Autodesk Inventor part; units mm, degrees
(part 2 of 2)
  line L320 (-21.6501, 50.3257) -> (-21.6501, 48.006)
  line L321 (-22.7741, 46.882) -> (-22.7741, 51.4497)
  line L322 (-19.4696, 52.5096) -> (-19.4696, 51.4497)
  line L323 (-13.5344, 50.3565) -> (-13.5344, 48.0368)
  line L324 (-15.3794, 53.4802) -> (-9.591, 53.4802)
  line L325 (-11.2436, 52.5096) -> (-11.2436, 51.4805)
  line L326 (-17.5447, 51.4497) -> (-17.5447, 46.882)
  line L327 (-14.6585, 46.9128) -> (-14.6585, 51.4805)
  line L328 (-14.6585, 51.4805) -> (-12.4852, 51.4805)
  line L329 (-12.4852, 51.4805) -> (-12.4852, 52.5096)
  line L330 (-9.591, 53.4802) -> (-9.591, 52.5096)
  line L331 (-9.591, 52.5096) -> (-11.2436, 52.5096)
  line L332 (-10.5531, 50.3565) -> (-13.5344, 50.3565)
  line L333 (-11.2436, 51.4805) -> (-9.429, 51.4805)
  line L334 (-13.5344, 48.0368) -> (-10.5531, 48.0368)
  line L335 (-9.429, 46.9128) -> (-14.6585, 46.9128)
  line L336 (-9.429, 51.4805) -> (-9.429, 46.9128)
  line L337 (-10.5531, 48.0368) -> (-10.5531, 50.3565)
  line L338 (-88.5687, 43.9647) -> (-88.5687, 42.994)
  line L339 (-88.5687, 42.994) -> (-86.5536, 42.994)
  line L340 (-92.6408, 44.9353) -> (-85.6563, 44.9353)
  line L341 (-87.6776, 41.87) -> (-90.659, 41.87)
  line L342 (-91.783, 42.994) -> (-89.7466, 42.994)
  line L343 (-87.6776, 39.5503) -> (-87.6776, 41.87)
  line L344 (-86.5536, 42.994) -> (-86.5536, 38.4263)
  line L345 (-90.659, 41.87) -> (-90.659, 39.5503)
  line L346 (-90.659, 39.5503) -> (-87.6776, 39.5503)
  line L347 (-86.5536, 38.4263) -> (-91.783, 38.4263)
  line L348 (-91.783, 38.4263) -> (-91.783, 42.994)
  line L349 (-89.7466, 42.994) -> (-89.7466, 43.9647)
  line L350 (-87.5813, 50.5629) -> (-82.3518, 50.5629)
  line L351 (-83.4759, 49.4389) -> (-86.4572, 49.4389)
  line L352 (-86.4572, 49.4389) -> (-86.4572, 47.1192)
  line L353 (-85.6563, 45.9951) -> (-87.5813, 45.9951)
  line L354 (-86.4572, 47.1192) -> (-83.4759, 47.1192)
  line L355 (-81.6326, 43.9647) -> (-88.5687, 43.9647)
  line L356 (-84.5732, 45.9951) -> (-84.5732, 44.9353)
  line L357 (-81.6326, 44.9353) -> (-81.6326, 43.9647)
  line L358 (-84.5732, 44.9353) -> (-81.6326, 44.9353)
  line L359 (-82.3518, 45.9951) -> (-84.5732, 45.9951)
  line L360 (-83.4759, 47.1192) -> (-83.4759, 49.4389)
  line L361 (-82.3518, 50.5629) -> (-82.3518, 45.9951)
  line L362 (-85.6563, 44.9353) -> (-85.6563, 45.9951)
  line L363 (-91.5915, 47.0884) -> (-91.5915, 49.4081)
  line L364 (-89.7466, 43.9647) -> (-95.535, 43.9647)
  line L365 (-93.8823, 44.9353) -> (-93.8823, 45.9644)
  line L366 (-87.5813, 45.9951) -> (-87.5813, 50.5629)
  line L367 (-90.4675, 50.5321) -> (-90.4675, 45.9644)
  line L368 (-90.4675, 45.9644) -> (-92.6408, 45.9644)
  line L369 (-92.6408, 45.9644) -> (-92.6408, 44.9353)
  line L370 (-95.535, 43.9647) -> (-95.535, 44.9353)
  line L371 (-95.535, 44.9353) -> (-93.8823, 44.9353)
  line L372 (-94.5729, 47.0884) -> (-91.5915, 47.0884)
  line L373 (-93.8823, 45.9644) -> (-95.6969, 45.9644)
  line L374 (-91.5915, 49.4081) -> (-94.5729, 49.4081)
  line L375 (-95.6969, 50.5321) -> (-90.4675, 50.5321)
  line L376 (-95.6969, 45.9644) -> (-95.6969, 50.5321)
  line L377 (-94.5729, 49.4081) -> (-94.5729, 47.0884)
  line L378 (-45.9553, 42.018) -> (-40.7259, 42.018)
  line L379 (-41.8499, 40.894) -> (-44.8313, 40.894)
  line L380 (-44.8313, 40.894) -> (-44.8313, 38.5743)
  line L381 (-44.8313, 38.5743) -> (-41.8499, 38.5743)
  line L382 (-40.7259, 42.018) -> (-40.7259, 37.4503)
  line L383 (-45.9553, 37.4503) -> (-45.9553, 42.018)
  line L384 (-44.0304, 37.4503) -> (-45.9553, 37.4503)
  line L385 (-40.7259, 37.4503) -> (-42.9473, 37.4503)
  line L386 (-51.0148, 36.3904) -> (-44.0304, 36.3904)
  line L387 (-42.9473, 37.4503) -> (-42.9473, 36.3904)
  line L388 (-42.9473, 36.3904) -> (-40.0067, 36.3904)
  line L389 (-44.0304, 36.3904) -> (-44.0304, 37.4503)
  line L390 (-40.0067, 35.4198) -> (-46.9428, 35.4198)
  line L391 (-40.0067, 36.3904) -> (-40.0067, 35.4198)
  line L392 (-41.8499, 38.5743) -> (-41.8499, 40.894)
  line L393 (-48.8415, 37.4195) -> (-51.0148, 37.4195)
  line L394 (-51.0148, 37.4195) -> (-51.0148, 36.3904)
  line L395 (-48.1206, 35.4198) -> (-53.909, 35.4198)
  line L396 (-52.2564, 36.3904) -> (-52.2564, 37.4195)
  line L397 (-53.909, 35.4198) -> (-53.909, 36.3904)
  line L398 (-53.909, 36.3904) -> (-52.2564, 36.3904)
  line L399 (-52.9469, 38.5435) -> (-49.9656, 38.5435)
  line L400 (-52.2564, 37.4195) -> (-54.071, 37.4195)
  line L401 (-49.9656, 38.5435) -> (-49.9656, 40.8632)
  line L402 (-48.8415, 41.9872) -> (-48.8415, 37.4195)
  line L403 (-49.9656, 40.8632) -> (-52.9469, 40.8632)
  line L404 (-52.9469, 40.8632) -> (-52.9469, 38.5435)
  line L405 (-54.071, 41.9872) -> (-48.8415, 41.9872)
  line L406 (-54.071, 37.4195) -> (-54.071, 41.9872)
  line L407 (-44.9276, 29.8814) -> (-50.157, 29.8814)
  line L408 (-49.033, 31.0054) -> (-46.0516, 31.0054)
  line L409 (-46.0516, 31.0054) -> (-46.0516, 33.3251)
  line L410 (-44.9276, 34.4492) -> (-44.9276, 29.8814)
  line L411 (-46.9428, 34.4492) -> (-44.9276, 34.4492)
  line L412 (-46.0516, 33.3251) -> (-49.033, 33.3251)
  line L413 (-49.033, 33.3251) -> (-49.033, 31.0054)
  line L414 (-46.9428, 35.4198) -> (-46.9428, 34.4492)
  line L415 (-50.157, 29.8814) -> (-50.157, 34.4492)
  line L416 (-48.1206, 34.4492) -> (-48.1206, 35.4198)
  line L417 (-50.157, 34.4492) -> (-48.1206, 34.4492)
  line L418 (-14.9833, 42.018) -> (-9.7539, 42.018)
  line L419 (-10.8779, 40.894) -> (-13.8593, 40.894)
  line L420 (-13.8593, 40.894) -> (-13.8593, 38.5743)
  line L421 (-13.8593, 38.5743) -> (-10.8779, 38.5743)
  line L422 (-9.7539, 42.018) -> (-9.7539, 37.4503)
  line L423 (-14.9833, 37.4503) -> (-14.9833, 42.018)
  line L424 (-13.0584, 37.4503) -> (-14.9833, 37.4503)
  line L425 (-9.7539, 37.4503) -> (-11.9752, 37.4503)
  line L426 (-20.0428, 36.3904) -> (-13.0584, 36.3904)
  line L427 (-11.9752, 37.4503) -> (-11.9752, 36.3904)
  line L428 (-11.9752, 36.3904) -> (-9.0346, 36.3904)
  line L429 (-13.0584, 36.3904) -> (-13.0584, 37.4503)
  line L430 (-9.0346, 35.4198) -> (-15.9708, 35.4198)
  line L431 (-9.0346, 36.3904) -> (-9.0346, 35.4198)
  line L432 (-10.8779, 38.5743) -> (-10.8779, 40.894)
  line L433 (-17.8695, 37.4195) -> (-20.0428, 37.4195)
  line L434 (-20.0428, 37.4195) -> (-20.0428, 36.3904)
  line L435 (-17.1486, 35.4198) -> (-22.937, 35.4198)
  line L436 (-21.2844, 36.3904) -> (-21.2844, 37.4195)
  line L437 (-22.937, 35.4198) -> (-22.937, 36.3904)
  line L438 (-22.937, 36.3904) -> (-21.2844, 36.3904)
  line L439 (-21.9749, 38.5435) -> (-18.9936, 38.5435)
  line L440 (-21.2844, 37.4195) -> (-23.099, 37.4195)
  line L441 (-18.9936, 38.5435) -> (-18.9936, 40.8632)
  line L442 (-17.8695, 41.9872) -> (-17.8695, 37.4195)
  line L443 (-18.9936, 40.8632) -> (-21.9749, 40.8632)
  line L444 (-21.9749, 40.8632) -> (-21.9749, 38.5435)
  line L445 (-23.099, 41.9872) -> (-17.8695, 41.9872)
  line L446 (-23.099, 37.4195) -> (-23.099, 41.9872)
  line L447 (-13.9556, 29.8814) -> (-19.185, 29.8814)
  line L448 (-18.061, 31.0054) -> (-15.0796, 31.0054)
  line L449 (-15.0796, 31.0054) -> (-15.0796, 33.3251)
  line L450 (-13.9556, 34.4492) -> (-13.9556, 29.8814)
  line L451 (-15.9708, 34.4492) -> (-13.9556, 34.4492)
  line L452 (-15.0796, 33.3251) -> (-18.061, 33.3251)
  line L453 (-18.061, 33.3251) -> (-18.061, 31.0054)
  line L454 (-15.9708, 35.4198) -> (-15.9708, 34.4492)
  line L455 (-19.185, 29.8814) -> (-19.185, 34.4492)
  line L456 (-17.1486, 34.4492) -> (-17.1486, 35.4198)
  line L457 (-19.185, 34.4492) -> (-17.1486, 34.4492)
  line L458 (-31.75, 0) -> (-63.5, 0) construction
  line L459 (-31.75, 88.9) -> (0, 88.9) construction
  line L460 (-31.75, 0) -> (-31.75, 88.9) construction
  line L461 (-24.2924, 69.3883) -> (-29.5218, 69.3883)
  line L462 (-28.3978, 70.5123) -> (-25.4164, 70.5123)
  line L463 (-25.4164, 72.832) -> (-28.3978, 72.832)
  line L464 (-25.4164, 70.5123) -> (-25.4164, 72.832)
  line L465 (-26.2173, 73.956) -> (-24.2924, 73.956)
  line L466 (-24.2924, 73.956) -> (-24.2924, 69.3883)
  line L467 (-29.5218, 69.3883) -> (-29.5218, 73.956)
  line L468 (-29.5218, 73.956) -> (-27.3004, 73.956)
  line L469 (-28.3978, 72.832) -> (-28.3978, 70.5123)
  line L470 (-26.2173, 75.0159) -> (-26.2173, 73.956)
  line L471 (-27.3004, 73.956) -> (-27.3004, 75.0159)
  line L472 (-27.3004, 75.0159) -> (-30.241, 75.0159)
  line L473 (-30.241, 75.0159) -> (-30.241, 75.9864)
  line L474 (-23.3049, 75.9864) -> (-23.3049, 76.9571)
  line L475 (-23.3049, 76.9571) -> (-25.3201, 76.9571)
  line L476 (-30.241, 75.9864) -> (-23.3049, 75.9864)
  line L477 (-17.9913, 75.0159) -> (-17.9913, 73.9868)
  line L478 (-20.2821, 72.8628) -> (-20.2821, 70.5431)
  line L479 (-22.127, 75.9864) -> (-16.3387, 75.9864)
  line L480 (-16.3387, 75.9864) -> (-16.3387, 75.0159)
  line L481 (-16.3387, 75.0159) -> (-17.9913, 75.0159)
  line L482 (-17.3007, 72.8628) -> (-20.2821, 72.8628)
  line L483 (-21.4061, 69.4191) -> (-21.4061, 73.9868)
  line L484 (-17.3007, 70.5431) -> (-17.3007, 72.8628)
  line L485 (-20.2821, 70.5431) -> (-17.3007, 70.5431)
  line L486 (-16.1767, 69.4191) -> (-21.4061, 69.4191)
  line L487 (-16.1767, 73.9868) -> (-16.1767, 69.4191)
  line L488 (-17.9913, 73.9868) -> (-16.1767, 73.9868)
  line L489 (-25.3201, 81.5249) -> (-20.0906, 81.5249)
  line L490 (-20.0906, 81.5249) -> (-20.0906, 76.9571)
  line L491 (-25.3201, 76.9571) -> (-25.3201, 81.5249)
  line L492 (-21.2147, 80.4009) -> (-24.196, 80.4009)
  line L493 (-24.196, 80.4009) -> (-24.196, 78.0812)
  line L494 (-24.196, 78.0812) -> (-21.2147, 78.0812)
  line L495 (-21.2147, 78.0812) -> (-21.2147, 80.4009)
  line L496 (-19.2329, 73.9868) -> (-19.2329, 75.0159)
  line L497 (-21.4061, 73.9868) -> (-19.2329, 73.9868)
  line L498 (-22.127, 76.9571) -> (-22.127, 75.9864)
  line L499 (-20.0906, 76.9571) -> (-22.127, 76.9571)
  line L500 (-19.2329, 75.0159) -> (-26.2173, 75.0159)
  line L501 (-38.0615, 19.4598) -> (-32.8321, 19.4598)
  line L502 (-33.9561, 18.3357) -> (-36.9375, 18.3357)
  line L503 (-36.9375, 18.3357) -> (-36.9375, 16.0161)
  line L504 (-36.9375, 16.0161) -> (-33.9561, 16.0161)
  line L505 (-32.8321, 19.4598) -> (-32.8321, 14.892)
  line L506 (-38.0615, 14.892) -> (-38.0615, 19.4598)
  line L507 (-36.1366, 14.892) -> (-38.0615, 14.892)
  line L508 (-32.8321, 14.892) -> (-35.0534, 14.892)
  line L509 (-43.121, 13.8322) -> (-36.1366, 13.8322)
  line L510 (-35.0534, 14.892) -> (-35.0534, 13.8322)
  line L511 (-35.0534, 13.8322) -> (-32.1128, 13.8322)
  line L512 (-36.1366, 13.8322) -> (-36.1366, 14.892)
  line L513 (-32.1128, 12.8616) -> (-39.0489, 12.8616)
  line L514 (-32.1128, 13.8322) -> (-32.1128, 12.8616)
  line L515 (-33.9561, 16.0161) -> (-33.9561, 18.3357)
  line L516 (-40.9477, 14.8613) -> (-43.121, 14.8613)
  line L517 (-43.121, 14.8613) -> (-43.121, 13.8322)
  line L518 (-40.2268, 12.8616) -> (-46.0152, 12.8616)
  line L519 (-44.3625, 13.8322) -> (-44.3625, 14.8613)
  line L520 (-46.0152, 12.8616) -> (-46.0152, 13.8322)
  line L521 (-46.0152, 13.8322) -> (-44.3625, 13.8322)
  line L522 (-45.0531, 15.9853) -> (-42.0717, 15.9853)
  line L523 (-44.3625, 14.8613) -> (-46.1771, 14.8613)
  line L524 (-42.0717, 15.9853) -> (-42.0717, 18.305)
  line L525 (-40.9477, 19.429) -> (-40.9477, 14.8613)
  line L526 (-42.0717, 18.305) -> (-45.0531, 18.305)
  line L527 (-45.0531, 18.305) -> (-45.0531, 15.9853)
  line L528 (-46.1771, 19.429) -> (-40.9477, 19.429)
  line L529 (-46.1771, 14.8613) -> (-46.1771, 19.429)
  line L530 (-37.0338, 7.3232) -> (-42.2632, 7.3232)
  line L531 (-41.1392, 8.4472) -> (-38.1578, 8.4472)
  line L532 (-38.1578, 8.4472) -> (-38.1578, 10.7669)
  line L533 (-37.0338, 11.8909) -> (-37.0338, 7.3232)
  line L534 (-39.0489, 11.8909) -> (-37.0338, 11.8909)
  line L535 (-38.1578, 10.7669) -> (-41.1392, 10.7669)
  line L536 (-41.1392, 10.7669) -> (-41.1392, 8.4472)
  line L537 (-39.0489, 12.8616) -> (-39.0489, 11.8909)
  line L538 (-42.2632, 7.3232) -> (-42.2632, 11.8909)
  line L539 (-40.2268, 11.8909) -> (-40.2268, 12.8616)
  line L540 (-42.2632, 11.8909) -> (-40.2268, 11.8909)
  line L541 (-22.4246, 19.4981) -> (-17.1952, 19.4981)
  line L542 (-18.3192, 18.3741) -> (-21.3006, 18.3741)
  line L543 (-21.3006, 18.3741) -> (-21.3006, 16.0544)
  line L544 (-21.3006, 16.0544) -> (-18.3192, 16.0544)
  line L545 (-17.1952, 19.4981) -> (-17.1952, 14.9304)
  line L546 (-22.4246, 14.9304) -> (-22.4246, 19.4981)
  line L547 (-20.4997, 14.9304) -> (-22.4246, 14.9304)
  line L548 (-17.1952, 14.9304) -> (-19.4165, 14.9304)
  line L549 (-27.4841, 13.8705) -> (-20.4997, 13.8705)
  line L550 (-19.4165, 14.9304) -> (-19.4165, 13.8705)
  line L551 (-19.4165, 13.8705) -> (-16.4759, 13.8705)
  line L552 (-20.4997, 13.8705) -> (-20.4997, 14.9304)
  line L553 (-16.4759, 12.9) -> (-23.412, 12.9)
  line L554 (-16.4759, 13.8705) -> (-16.4759, 12.9)
  line L555 (-18.3192, 16.0544) -> (-18.3192, 18.3741)
  line L556 (-25.3108, 14.8996) -> (-27.4841, 14.8996)
  line L557 (-27.4841, 14.8996) -> (-27.4841, 13.8705)
  line L558 (-24.5899, 12.9) -> (-30.3783, 12.9)
  line L559 (-28.7257, 13.8705) -> (-28.7257, 14.8996)
  line L560 (-30.3783, 12.9) -> (-30.3783, 13.8705)
  line L561 (-30.3783, 13.8705) -> (-28.7257, 13.8705)
  line L562 (-29.4162, 16.0236) -> (-26.4349, 16.0236)
  line L563 (-28.7257, 14.8996) -> (-30.5403, 14.8996)
  line L564 (-26.4349, 16.0236) -> (-26.4349, 18.3433)
  line L565 (-25.3108, 19.4673) -> (-25.3108, 14.8996)
  line L566 (-26.4349, 18.3433) -> (-29.4162, 18.3433)
  line L567 (-29.4162, 18.3433) -> (-29.4162, 16.0236)
  line L568 (-30.5403, 19.4673) -> (-25.3108, 19.4673)
  line L569 (-30.5403, 14.8996) -> (-30.5403, 19.4673)
  line L570 (-21.3969, 7.3615) -> (-26.6263, 7.3615)
  line L571 (-25.5023, 8.4855) -> (-22.5209, 8.4855)
  line L572 (-22.5209, 8.4855) -> (-22.5209, 10.8052)
  line L573 (-21.3969, 11.9293) -> (-21.3969, 7.3615)
  line L574 (-23.412, 11.9293) -> (-21.3969, 11.9293)
  line L575 (-22.5209, 10.8052) -> (-25.5023, 10.8052)
  line L576 (-25.5023, 10.8052) -> (-25.5023, 8.4855)
  line L577 (-23.412, 12.9) -> (-23.412, 11.9293)
  line L578 (-26.6263, 7.3615) -> (-26.6263, 11.9293)
  line L579 (-24.5899, 11.9293) -> (-24.5899, 12.9)
  line L580 (-26.6263, 11.9293) -> (-24.5899, 11.9293)
  line L581 (-54.8737, 75.3003) -> (-59.8302, 75.3003)
  line L582 (-59.8302, 75.3003) -> (-59.8302, 76.3377)
  line L583 (-59.8302, 76.3377) -> (-57.9859, 76.3377)
  line L584 (-57.9859, 76.3377) -> (-57.9859, 83.1467)
  line L585 (-57.9859, 83.1467) -> (-59.8302, 83.1467)
  line L586 (-59.8302, 83.1467) -> (-59.8302, 84.0771)
  spline S0 degree 2 poles (-59.8302, 84.0771) (-58.7846, 84.0771) (-57.7966, 84.6699) (-57.7307, 85.4932) knots 0 0 0 1 2 2 2
  line L587 (-57.7307, 85.4932) -> (-56.6768, 85.4932)
  line L588 (-56.6768, 85.4932) -> (-56.6768, 76.3377)
  line L589 (-56.6768, 76.3377) -> (-54.8737, 76.3377)
  line L590 (-54.8737, 76.3377) -> (-54.8737, 75.3003)
  spline S1 degree 2 poles (-46.6815, 80.3803) (-46.6815, 77.6468) (-48.2705, 75.0862) (-49.9255, 75.0862) knots 0 0 0 1 2 2 2
  spline S2 degree 2 poles (-49.9255, 75.0862) (-51.6051, 75.0862) (-53.1776, 77.6962) (-53.1776, 80.3721) knots 0 0 0 1 2 2 2
  spline S3 degree 2 poles (-53.1776, 80.3721) (-53.1776, 83.122) (-51.5886, 85.6661) (-49.9255, 85.6661) knots 0 0 0 1 2 2 2
  spline S4 degree 2 poles (-49.9255, 85.6661) (-48.2541, 85.6661) (-46.6815, 83.0314) (-46.6815, 80.3803) knots 0 0 0 1 2 2 2
  spline S5 degree 2 poles (-48.427, 77.2845) (-48.2294, 77.7868) (-48.0647, 79.3347) (-48.0647, 80.3803) knots 0 0 0 1 2 2 2
  spline S6 degree 2 poles (-48.0647, 80.3803) (-48.0647, 81.4259) (-48.2294, 82.9656) (-48.4352, 83.4843) knots 0 0 0 1 2 2 2
  spline S7 degree 2 poles (-48.4352, 83.4843) (-48.641, 84.003) (-49.3573, 84.5382) (-49.9255, 84.5382) knots 0 0 0 1 2 2 2
  spline S8 degree 2 poles (-49.9255, 84.5382) (-50.4936, 84.5382) (-51.2263, 84.003) (-51.4404, 83.4678) knots 0 0 0 1 2 2 2
  spline S9 degree 2 poles (-51.4404, 83.4678) (-51.6462, 82.9491) (-51.7944, 81.3683) (-51.7944, 80.3721) knots 0 0 0 1 2 2 2
  spline S10 degree 2 poles (-51.7944, 80.3721) (-51.7944, 79.3017) (-51.6627, 77.8691) (-51.4486, 77.3092) knots 0 0 0 1 2 2 2
  spline S11 degree 2 poles (-51.4486, 77.3092) (-51.251, 76.7823) (-50.5183, 76.2142) (-49.9255, 76.2142) knots 0 0 0 1 2 2 2
  spline S12 degree 2 poles (-49.9255, 76.2142) (-49.3656, 76.2142) (-48.6328, 76.7494) (-48.427, 77.2845) knots 0 0 0 1 2 2 2
  line L591 (-8.6263, 13.7693) -> (-3.6698, 13.7693)
  line L592 (-3.6698, 13.7693) -> (-3.6698, 12.7319)
  line L593 (-3.6698, 12.7319) -> (-5.5141, 12.7319)
  line L594 (-5.5141, 12.7319) -> (-5.5141, 5.9229)
  line L595 (-5.5141, 5.9229) -> (-3.6698, 5.9229)
  line L596 (-3.6698, 5.9229) -> (-3.6698, 4.9926)
  spline S13 degree 2 poles (-3.6698, 4.9926) (-4.7154, 4.9926) (-5.7034, 4.3998) (-5.7693, 3.5764) knots 0 0 0 1 2 2 2
  line L597 (-5.7693, 3.5764) -> (-6.8232, 3.5764)
  line L598 (-6.8232, 3.5764) -> (-6.8232, 12.7319)
  line L599 (-6.8232, 12.7319) -> (-8.6263, 12.7319)
  line L600 (-8.6263, 12.7319) -> (-8.6263, 13.7693)
  spline S14 degree 2 poles (-16.8185, 8.6893) (-16.8185, 11.4228) (-15.2295, 13.9834) (-13.5745, 13.9834) knots 0 0 0 1 2 2 2
  spline S15 degree 2 poles (-13.5745, 13.9834) (-11.8949, 13.9834) (-10.3224, 11.3734) (-10.3224, 8.6976) knots 0 0 0 1 2 2 2
  spline S16 degree 2 poles (-10.3224, 8.6976) (-10.3224, 5.9476) (-11.9114, 3.4035) (-13.5745, 3.4035) knots 0 0 0 1 2 2 2
  spline S17 degree 2 poles (-13.5745, 3.4035) (-15.2459, 3.4035) (-16.8185, 6.0382) (-16.8185, 8.6893) knots 0 0 0 1 2 2 2
  spline S18 degree 2 poles (-15.073, 11.7851) (-15.2706, 11.2829) (-15.4353, 9.735) (-15.4353, 8.6893) knots 0 0 0 1 2 2 2
  spline S19 degree 2 poles (-15.4353, 8.6893) (-15.4353, 7.6437) (-15.2706, 6.1041) (-15.0648, 5.5854) knots 0 0 0 1 2 2 2
  spline S20 degree 2 poles (-15.0648, 5.5854) (-14.859, 5.0667) (-14.1427, 4.5315) (-13.5745, 4.5315) knots 0 0 0 1 2 2 2
  spline S21 degree 2 poles (-13.5745, 4.5315) (-13.0064, 4.5315) (-12.2737, 5.0667) (-12.0596, 5.6018) knots 0 0 0 1 2 2 2
  spline S22 degree 2 poles (-12.0596, 5.6018) (-11.8538, 6.1205) (-11.7056, 7.7013) (-11.7056, 8.6976) knots 0 0 0 1 2 2 2
  spline S23 degree 2 poles (-11.7056, 8.6976) (-11.7056, 9.7679) (-11.8373, 11.2005) (-12.0514, 11.7604) knots 0 0 0 1 2 2 2
  spline S24 degree 2 poles (-12.0514, 11.7604) (-12.249, 12.2873) (-12.9817, 12.8554) (-13.5745, 12.8554) knots 0 0 0 1 2 2 2
  spline S25 degree 2 poles (-13.5745, 12.8554) (-14.1344, 12.8554) (-14.8672, 12.3203) (-15.073, 11.7851) knots 0 0 0 1 2 2 2
  line L601 (-8.6263, 13.7693) -> (-3.6698, 13.7693)
  line L602 (-3.6698, 13.7693) -> (-3.6698, 12.7319)
  line L603 (-3.6698, 12.7319) -> (-5.5141, 12.7319)
  line L604 (-5.5141, 12.7319) -> (-5.5141, 5.9229)
  line L605 (-5.5141, 5.9229) -> (-3.6698, 5.9229)
  line L606 (-3.6698, 5.9229) -> (-3.6698, 4.9926)
  spline S26 degree 2 poles (-3.6698, 4.9926) (-4.7154, 4.9926) (-5.7034, 4.3998) (-5.7693, 3.5764) knots 0 0 0 1 2 2 2
  line L607 (-5.7693, 3.5764) -> (-6.8232, 3.5764)
  line L608 (-6.8232, 3.5764) -> (-6.8232, 12.7319)
  line L609 (-6.8232, 12.7319) -> (-8.6263, 12.7319)
  line L610 (-8.6263, 12.7319) -> (-8.6263, 13.7693)
  spline S27 degree 2 poles (-16.8185, 8.6893) (-16.8185, 11.4228) (-15.2295, 13.9834) (-13.5745, 13.9834) knots 0 0 0 1 2 2 2
  spline S28 degree 2 poles (-13.5745, 13.9834) (-11.8949, 13.9834) (-10.3224, 11.3734) (-10.3224, 8.6976) knots 0 0 0 1 2 2 2
  spline S29 degree 2 poles (-10.3224, 8.6976) (-10.3224, 5.9476) (-11.9114, 3.4035) (-13.5745, 3.4035) knots 0 0 0 1 2 2 2
  spline S30 degree 2 poles (-13.5745, 3.4035) (-15.2459, 3.4035) (-16.8185, 6.0382) (-16.8185, 8.6893) knots 0 0 0 1 2 2 2
  spline S31 degree 2 poles (-15.073, 11.7851) (-15.2706, 11.2829) (-15.4353, 9.735) (-15.4353, 8.6893) knots 0 0 0 1 2 2 2
  spline S32 degree 2 poles (-15.4353, 8.6893) (-15.4353, 7.6437) (-15.2706, 6.1041) (-15.0648, 5.5854) knots 0 0 0 1 2 2 2
  spline S33 degree 2 poles (-15.0648, 5.5854) (-14.859, 5.0667) (-14.1427, 4.5315) (-13.5745, 4.5315) knots 0 0 0 1 2 2 2
  spline S34 degree 2 poles (-13.5745, 4.5315) (-13.0064, 4.5315) (-12.2737, 5.0667) (-12.0596, 5.6018) knots 0 0 0 1 2 2 2
  spline S35 degree 2 poles (-12.0596, 5.6018) (-11.8538, 6.1205) (-11.7056, 7.7013) (-11.7056, 8.6976) knots 0 0 0 1 2 2 2
  spline S36 degree 2 poles (-11.7056, 8.6976) (-11.7056, 9.7679) (-11.8373, 11.2005) (-12.0514, 11.7604) knots 0 0 0 1 2 2 2
  spline S37 degree 2 poles (-12.0514, 11.7604) (-12.249, 12.2873) (-12.9817, 12.8554) (-13.5745, 12.8554) knots 0 0 0 1 2 2 2
  spline S38 degree 2 poles (-13.5745, 12.8554) (-14.1344, 12.8554) (-14.8672, 12.3203) (-15.073, 11.7851) knots 0 0 0 1 2 2 2
  line L611 (-54.8737, 75.3003) -> (-59.8302, 75.3003)
  line L612 (-59.8302, 75.3003) -> (-59.8302, 76.3377)
  line L613 (-59.8302, 76.3377) -> (-57.9859, 76.3377)
  line L614 (-57.9859, 76.3377) -> (-57.9859, 83.1467)
  line L615 (-57.9859, 83.1467) -> (-59.8302, 83.1467)
  line L616 (-59.8302, 83.1467) -> (-59.8302, 84.0771)
  spline S39 degree 2 poles (-59.8302, 84.0771) (-58.7846, 84.0771) (-57.7966, 84.6699) (-57.7307, 85.4932) knots 0 0 0 1 2 2 2
  line L617 (-57.7307, 85.4932) -> (-56.6768, 85.4932)
  line L618 (-56.6768, 85.4932) -> (-56.6768, 76.3377)
  line L619 (-56.6768, 76.3377) -> (-54.8737, 76.3377)
  line L620 (-54.8737, 76.3377) -> (-54.8737, 75.3003)
  spline S40 degree 2 poles (-46.6815, 80.3803) (-46.6815, 77.6468) (-48.2705, 75.0862) (-49.9255, 75.0862) knots 0 0 0 1 2 2 2
  spline S41 degree 2 poles (-49.9255, 75.0862) (-51.6051, 75.0862) (-53.1776, 77.6962) (-53.1776, 80.3721) knots 0 0 0 1 2 2 2
  spline S42 degree 2 poles (-53.1776, 80.3721) (-53.1776, 83.122) (-51.5886, 85.6661) (-49.9255, 85.6661) knots 0 0 0 1 2 2 2
  spline S43 degree 2 poles (-49.9255, 85.6661) (-48.2541, 85.6661) (-46.6815, 83.0314) (-46.6815, 80.3803) knots 0 0 0 1 2 2 2
  spline S44 degree 2 poles (-48.427, 77.2845) (-48.2294, 77.7868) (-48.0647, 79.3347) (-48.0647, 80.3803) knots 0 0 0 1 2 2 2
  spline S45 degree 2 poles (-48.0647, 80.3803) (-48.0647, 81.4259) (-48.2294, 82.9656) (-48.4352, 83.4843) knots 0 0 0 1 2 2 2
  spline S46 degree 2 poles (-48.4352, 83.4843) (-48.641, 84.003) (-49.3573, 84.5382) (-49.9255, 84.5382) knots 0 0 0 1 2 2 2
  spline S47 degree 2 poles (-49.9255, 84.5382) (-50.4936, 84.5382) (-51.2263, 84.003) (-51.4404, 83.4678) knots 0 0 0 1 2 2 2
  spline S48 degree 2 poles (-51.4404, 83.4678) (-51.6462, 82.9491) (-51.7944, 81.3683) (-51.7944, 80.3721) knots 0 0 0 1 2 2 2
  spline S49 degree 2 poles (-51.7944, 80.3721) (-51.7944, 79.3017) (-51.6627, 77.8691) (-51.4486, 77.3092) knots 0 0 0 1 2 2 2
  spline S50 degree 2 poles (-51.4486, 77.3092) (-51.251, 76.7823) (-50.5183, 76.2142) (-49.9255, 76.2142) knots 0 0 0 1 2 2 2
  spline S51 degree 2 poles (-49.9255, 76.2142) (-49.3656, 76.2142) (-48.6328, 76.7494) (-48.427, 77.2845) knots 0 0 0 1 2 2 2
  point P0 (-38.5048, 75.5531)
  point P1 (-53.7479, 68.8958)
  point P2 (-9.7521, 20.0042)
  point P3 (-41.8348, 101.4209)
  point P4 (-40.4883, 75.5012)
  point P5 (-53.7479, 68.8958)
  point P6 (-9.7521, 20.0042)
  point P7 (-1, 6.9835)
  point P8 (-31.7444, 28.893)
  point P9 (-31.7444, 28.893)
  point P10 (-47.236, 52.9949)
  point P11 (-47.236, 52.9949)
  point P12 (-31.7444, 60.007)
  point P13 (-31.7444, 60.007)
  point P14 (-31.7444, 60.007)
  point P15 (-31.7444, 28.893)
  point P16 (-16.264, 52.9949)
  point P17 (-47.236, 35.9051)
  point P18 (-16.264, 35.9051)
  point P19 (-16.264, 52.9949)
  point P20 (-16.264, 52.9949)
  point P21 (-88.862, 44.45)
  point P22 (-88.862, 44.45)
  point P23 (-47.236, 35.9051)
  point P24 (-47.236, 35.9051)
  point P25 (-16.264, 35.9051)
  point P26 (-16.264, 35.9051)
  point P27 (-23.0117, 75.5012)
  point P28 (-23.0117, 75.5012)
  point P29 (-27.964, 75.5012)
  point P30 (-39.3422, 13.3469)
  point P31 (-23.7053, 13.3852)
  point P32 (-39.3422, 13.3469)
  point P33 (-39.3422, 13.3469)
  point P34 (-23.7053, 13.3852)
  point P35 (-23.7053, 13.3852)
  dimension "d155" = 8.4153
  dimension "d157" = 0.508
  dimension "d158" = 4.5466
  dimension "d159" = 0.508
  dimension "d160" = 4.5466
  constraints: 1132 end point, 50 parallel, 20 perpendicular, 14 horizontal, 3 midpoint, 3 symmetric about line, 1 vertical, 14 other
  measures "d155" distance of L174.end L172.start
  measures "d157" distance between parallel lines of L7 L173
  measures "d158" distance from line of point (-1, 6.983) L172
  measures "d159" distance between parallel lines of L6 L168
  measures "d160" distance between parallel lines of L4 L171
extrude "Extrusion20" add sketch "Sketch17" along normal blind 0.4 contours L48 L49 L73 L71 L76 L69 L86 L79 L85 L67 L62 L68 L84 L80 L87 L77 L82 L60 L55 L61 L81 L78 L83 L70 L75 L72 L74 L50 | L88 L89 L113 L111 L116 L109 L126 L119 L125 L107 L102 L108 L124 L120 L127 L117 L122 L100 L95 L101 L121 L118 L123 L110 L115 L112 L114 L90 | L128 L129 L153 L151 L156 L149 L166 L159 L165 L147 L142 L148 L164 L160 L167 L157 L162 L140 L135 L141 L161 L158 L163 L150 L155 L152 L154 L130 | L177 L183 L184 L187 L188 L189 L192 L190 L191 L207 L205 L206 L215 L214 L195 L196 L197 L193 L204 L203 L202 L199 L213 L212 L216 L186 L181 L182 | L218 L230 L227 L226 L228 L235 L224 L232 L234 L253 L254 L255 L246 L245 L221 L242 L241 L231 L256 L243 L240 L236 L252 L251 L244 L225 L222 L233 | L258 L270 L267 L266 L268 L275 L264 L272 L274 L293 L294 L295 L286 L285 L261 L282 L281 L271 L296 L283 L280 L276 L292 L291 L284 L265 L262 L273 | L298 L299 L304 L307 L308 L302 L309 L324 L330 L331 L325 L333 L336 L335 L327 L328 L329 L300 L322 L313 L326 L310 L321 L319 L316 L318 L317 L315 | L378 L382 L385 L387 L388 L391 L390 L414 L411 L410 L407 L415 L417 L416 L395 L397 L398 L396 L400 L406 L405 L402 L393 L394 L386 L389 L384 L383 | L418 L422 L425 L427 L428 L431 L430 L454 L451 L450 L447 L455 L457 L456 L435 L437 L438 L436 L440 L446 L445 L442 L433 L434 L426 L429 L424 L423 | L461 L467 L468 L471 L472 L473 L476 L474 L475 L491 L489 L490 L499 L498 L479 L480 L481 L477 L488 L487 L486 L483 L497 L496 L500 L470 L465 L466 | L501 L505 L508 L510 L511 L514 L513 L537 L534 L533 L530 L538 L540 L539 L518 L520 L521 L519 L523 L529 L528 L525 L516 L517 L509 L512 L507 L506 | L541 L545 L548 L550 L551 L554 L553 L577 L574 L573 L570 L578 L580 L579 L558 L560 L561 L559 L563 L569 L568 L565 L556 L557 L549 L552 L547 L546 | L581 L582 L583 L584 L585 L586 S0 L587 L588 L589 L590 | S1 S2 S3 S4 | L591 L592 L593 L594 L595 L596 S13 L597 L598 L599 L600 | S14 S15 S16 S17 bodies 2
sketch "Sketch18" plane through (0, 0, -0.2) normal (0, 0, -1) x (-1, 0, 0)
  line L0 (0, 0) -> (-63.5, 0)
  line L1 (-63.5, 0) -> (-63.5, 88.9)
  line L2 (-63.5, 88.9) -> (0, 88.9)
  line L3 (0, 88.9) -> (0, 0)
  constraints: 8 end point, 2 parallel, 1 horizontal, 1 perpendicular
extrude "Extrusion21" add sketch "Sketch18" along normal blind 0.4 bodies 3
fillet "Fillet2" radius 3.175 8 edges at (63.5, 0, 0.2) (63.5, 88.9, 0.2) (0, 0, 0.2) (0, 88.9, 0.2) (63.5, 0, -0.3) (63.5, 88.9, -0.3) (0, 0, -0.3) (0, 88.9, -0.3)
extrude "Extrusion22" cut sketch "Sketch17" along normal blind 0.4 contours L48 L49 L73 L71 L76 L69 L86 L79 L85 L67 L62 L68 L84 L80 L87 L77 L82 L60 L55 L61 L81 L78 L83 L70 L75 L72 L74 L50 | L88 L89 L113 L111 L116 L109 L126 L119 L125 L107 L102 L108 L124 L120 L127 L117 L122 L100 L95 L101 L121 L118 L123 L110 L115 L112 L114 L90 | L128 L129 L153 L151 L156 L149 L166 L159 L165 L147 L142 L148 L164 L160 L167 L157 L162 L140 L135 L141 L161 L158 L163 L150 L155 L152 L154 L130 | L177 L183 L184 L187 L188 L189 L192 L190 L191 L207 L205 L206 L215 L214 L195 L196 L197 L193 L204 L203 L202 L199 L213 L212 L216 L186 L181 L182 | L218 L230 L227 L226 L228 L235 L224 L232 L234 L253 L254 L255 L246 L245 L221 L242 L241 L231 L256 L243 L240 L236 L252 L251 L244 L225 L222 L233 | L258 L270 L267 L266 L268 L275 L264 L272 L274 L293 L294 L295 L286 L285 L261 L282 L281 L271 L296 L283 L280 L276 L292 L291 L284 L265 L262 L273 | L298 L299 L304 L307 L308 L302 L309 L324 L330 L331 L325 L333 L336 L335 L327 L328 L329 L300 L322 L313 L326 L310 L321 L319 L316 L318 L317 L315 | L378 L382 L385 L387 L388 L391 L390 L414 L411 L410 L407 L415 L417 L416 L395 L397 L398 L396 L400 L406 L405 L402 L393 L394 L386 L389 L384 L383 | L418 L422 L425 L427 L428 L431 L430 L454 L451 L450 L447 L455 L457 L456 L435 L437 L438 L436 L440 L446 L445 L442 L433 L434 L426 L429 L424 L423 | L461 L467 L468 L471 L472 L473 L476 L474 L475 L491 L489 L490 L499 L498 L479 L480 L481 L477 L488 L487 L486 L483 L497 L496 L500 L470 L465 L466 | L501 L505 L508 L510 L511 L514 L513 L537 L534 L533 L530 L538 L540 L539 L518 L520 L521 L519 L523 L529 L528 L525 L516 L517 L509 L512 L507 L506 | L541 L545 L548 L550 L551 L554 L553 L577 L574 L573 L570 L578 L580 L579 L558 L560 L561 L559 L563 L569 L568 L565 L556 L557 L549 L552 L547 L546 | L581 L582 L583 L584 L585 L586 S0 L587 L588 L589 L590 | S1 S2 S3 S4 | L591 L592 L593 L594 L595 L596 S13 L597 L598 L599 L600 | S14 S15 S16 S17 bodies 3
